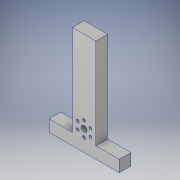
# Autodesk Inventor part: Motor Block
Saved by Autodesk Inventor 2019 (Build 230136000, 136)
## iProperties
Created: 2019-03-05
Part Number: Motor Block
Material: Aluminum 6061
Document SubType Name: Modeling
Designer: Delta
Density: 2.7 g/cm^3
Appearance: Aluminum - Flat
Mass: 116.194 g
Surface Area: 125.486 cm^2
Volume: 43.0347 cm^3
Author: Delta
Autodesk Inventor part; units mm, degrees
ref_plane "YZ Plane" through (0, 0, 0) normal (1, 0, 0) x (0, 1, 0)
ref_plane "XZ Plane" through (0, 0, 0) normal (0, 1, 0) x (-1, 0, 0)
ref_plane "XY Plane" through (0, 0, 0) normal (0, 0, 1) x (1, 0, 0)
sketch "Sketch1" plane through (0, 0, 0) normal (0, 0, 1) x (1, 0, 0)
  line L0 (0, 0) -> (25.4, 0)
  line L1 (25.4, 0) -> (25.4, 111.125)
  line L2 (25.4, 111.125) -> (0, 111.125)
  line L3 (0, 111.125) -> (0, 0)
  dimension "d0" = 25.4
  dimension "d1" = 111.125
  constraints: 8 end point, 2 parallel, 1 horizontal, 1 perpendicular
  measures "d0" distance of L2.end L1.end
  measures "d1" distance of L1.end L0.end
extrude "Extrusion1" add sketch "Sketch1" along normal blind 12.7
sketch "Sketch2" plane through (0, 0, 12.7) normal (0, 0, 1) x (1, 0, 0)
  line L0 (25.4, 111.125) -> (0, 111.125) projected
  line L1 (25.4, 0) -> (25.4, 111.125) projected
  point P0 (0, 0)
  point P1 (12.7, 22.225)
  dimension "d4" = 88.9
  dimension "d5" = 25.4
  dimension "d6" = 12.7
  measures "d4" distance from line of point (12.7, 22.225) L0
  measures "d5" distance of L0.start L0.end
  measures "d6" distance from line of L1 point (12.7, 22.225)
hole "Hole1" at (12.7, 22.225, 12.7) direction (0, 0, -1) diameter 6.35 end through all
sketch "Sketch3" plane through (0, 0, 12.7) normal (0, 0, 1) x (1, 0, 0)
  circle A0 centre (12.7, 22.225) radius 3.175 projected
  line L0 (0, 111.125) -> (0, 0) projected
  point P0 (12.7, 30.226)
  dimension "d14" = 8.001
  dimension "d15" = 12.7
  measures "d14" distance of A0.centre point (12.7, 30.226)
  measures "d15" distance from line of L0 point (12.7, 30.226)
hole "Hole2" at (12.7, 30.226, 12.7) direction (0, 0, -1) diameter 3.175 end through all
pattern_circular "Circular Pattern1" count 6 over 360 about axis through (12.7, 22.225, -101.9962) along (0, 0, 1) of "Hole2"
sketch "Sketch5" plane through (25.4, 0, 0) normal (1, 0, 0) x (0, 0, -1)
  line L0 (0, 0) -> (-12.7, 0) projected
  line L1 (-12.7, 12.6365) -> (-12.7, 15.8115) projected
  line L2 (0, 0) -> (-12.7, 0)
  line L3 (-12.7, 0) -> (-12.7, 12.7)
  line L4 (-12.7, 12.7) -> (0, 12.7)
  line L5 (0, 12.7) -> (0, 0)
  dimension "d26" = 12.7
  constraints: 8 end point, 2 parallel, 1 horizontal, 1 perpendicular, 1 point on line
  measures "d26" distance of L2.end L3.end
extrude "Extrusion2" add sketch "Sketch5" along normal blind 25.4
ref_plane "Work Plane1" through (12.7, 111.125, 12.7) normal (1, 0, 0) x (0, 0, -1)
mirror "Mirror1" about plane through (12.7, 111.125, 12.7) normal (1, 0, 0) of "Extrusion2"
equation "\"d6\" = 0.5 * d5"
body "Solid1"
